Autodesk Fusion 360 part; units mm, degrees
note: some values were not read from the file. Chosen so that the rebuilt part matches the saved one: a direction. Set by a fixed rule: which sketch regions a step uses.
(part 3 of 6)
  spline S31 degree 5 poles (7.4784, -26.4341) (7.4757, -26.4291) (7.4705, -26.4191) (7.463, -26.4039) (7.4538, -26.3832) (7.4432, -26.357) (7.4334, -26.3303) (7.4239, -26.3035) (7.4148, -26.2765) (7.4058, -26.2495) (7.3969, -26.2223) (7.3883, -26.1951) (7.38, -26.1677) (7.3721, -26.1402) (7.3644, -26.1125) (7.3571, -26.0846) (7.3501, -26.0566) (7.3434, -26.0285) (7.3368, -26.0003) (7.3304, -25.9721) (7.3243, -25.9437) (7.3183, -25.9153) (7.3126, -25.8867) (7.307, -25.8581) (7.3017, -25.8294) (7.2966, -25.8006) (7.2917, -25.7717) (7.287, -25.7427) (7.2825, -25.7137) (7.2782, -25.6845) (7.2741, -25.6553) (7.2701, -25.6261) (7.2663, -25.5967) (7.2627, -25.5673) (7.2593, -25.5379) (7.256, -25.5083) (7.253, -25.4787) (7.2501, -25.4491) (7.2474, -25.4193) (7.2448, -25.3895) (7.2424, -25.3597) (7.2402, -25.3298) (7.2381, -25.2998) (7.2362, -25.2698) (7.2345, -25.2397) (7.2329, -25.2096) (7.2315, -25.1794) (7.2302, -25.1492) (7.2291, -25.1189) (7.2282, -25.0885) (7.2274, -25.0581) (7.2267, -25.0277) (7.2263, -24.9972) (7.2259, -24.9667) (7.2257, -24.9361) (7.2257, -24.9055) (7.2258, -24.8748) (7.2261, -24.8441) (7.2265, -24.8134) (7.227, -24.7826) (7.2278, -24.7517) (7.2286, -24.7208) (7.2296, -24.6899) (7.2307, -24.659) (7.232, -24.628) (7.2335, -24.5969) (7.235, -24.5659) (7.2367, -24.5348) (7.2386, -24.5036) (7.2406, -24.4724) (7.2427, -24.4412) (7.2445, -24.4162) (7.2459, -24.3975) (7.2469, -24.3849) (7.2474, -24.3787) knots 0 0 0 0 0 0 0.01428571 0.02857143 0.04285714 0.05714286 0.07142857 0.08571429 0.1 0.11428571 0.12857143 0.14285714 0.15714286 0.17142857 0.18571429 0.2 0.21428571 0.22857143 0.24285714 0.25714286 0.27142857 0.28571429 0.3 0.31428571 0.32857143 0.34285714 0.35714286 0.37142857 0.38571429 0.4 0.41428571 0.42857143 0.44285714 0.45714286 0.47142857 0.48571429 0.5 0.51428571 0.52857143 0.54285714 0.55714286 0.57142857 0.58571429 0.6 0.61428571 0.62857143 0.64285714 0.65714286 0.67142857 0.68571429 0.7 0.71428571 0.72857143 0.74285714 0.75714286 0.77142857 0.78571429 0.8 0.81428571 0.82857143 0.84285714 0.85714286 0.87142857 0.88571429 0.9 0.91428571 0.92857143 0.94285714 0.95714286 0.97142857 0.98571429 1 1 1 1 1 1
  line L31 (7.4784, -26.4341) -> (7.7091, -26.8632)
  arc A63 (7.6692, -26.9982) -> (7.7091, -26.8632) centre (7.621, -26.9106) ccw
  arc A64 (7.6692, -26.9982) -> (6.7944, -27.5287) centre (13.5, -37.5997) ccw
  arc A65 (6.6562, -27.5017) -> (6.7944, -27.5287) centre (6.7389, -27.4455) ccw
  line L32 (6.6562, -27.5017) -> (6.3823, -27.0988)
  spline S32 degree 5 poles (6.3823, -27.0988) (6.3792, -27.0941) (6.3727, -27.0848) (6.3626, -27.0712) (6.3486, -27.0534) (6.3302, -27.0319) (6.3112, -27.0109) (6.2917, -26.9901) (6.2721, -26.9695) (6.2522, -26.949) (6.2322, -26.9287) (6.2121, -26.9084) (6.1916, -26.8884) (6.1709, -26.8686) (6.1498, -26.849) (6.1285, -26.8297) (6.1069, -26.8105) (6.0851, -26.7916) (6.0632, -26.7727) (6.041, -26.754) (6.0188, -26.7354) (5.9963, -26.717) (5.9736, -26.6987) (5.9508, -26.6806) (5.9278, -26.6626) (5.9046, -26.6447) (5.8812, -26.627) (5.8577, -26.6095) (5.8341, -26.5921) (5.8102, -26.5748) (5.7863, -26.5576) (5.7621, -26.5405) (5.7379, -26.5236) (5.7135, -26.5068) (5.6889, -26.4902) (5.6642, -26.4737) (5.6394, -26.4573) (5.6144, -26.441) (5.5893, -26.4248) (5.5641, -26.4088) (5.5387, -26.3929) (5.5132, -26.3771) (5.4876, -26.3614) (5.4619, -26.3458) (5.436, -26.3304) (5.41, -26.315) (5.3839, -26.2998) (5.3577, -26.2847) (5.3313, -26.2698) (5.3048, -26.2549) (5.2783, -26.2401) (5.2516, -26.2255) (5.2248, -26.211) (5.1978, -26.1966) (5.1708, -26.1823) (5.1437, -26.1681) (5.1164, -26.154) (5.0891, -26.1401) (5.0616, -26.1262) (5.034, -26.1125) (5.0064, -26.0988) (4.9786, -26.0853) (4.9507, -26.0719) (4.9227, -26.0586) (4.8947, -26.0454) (4.8665, -26.0323) (4.8382, -26.0194) (4.8098, -26.0065) (4.7814, -25.9937) (4.7528, -25.9811) (4.7241, -25.9686) (4.7011, -25.9586) (4.6838, -25.9512) (4.6723, -25.9463) (4.6665, -25.9438) knots 0 0 0 0 0 0 0.01428571 0.02857143 0.04285714 0.05714286 0.07142857 0.08571429 0.1 0.11428571 0.12857143 0.14285714 0.15714286 0.17142857 0.18571429 0.2 0.21428571 0.22857143 0.24285714 0.25714286 0.27142857 0.28571429 0.3 0.31428571 0.32857143 0.34285714 0.35714286 0.37142857 0.38571429 0.4 0.41428571 0.42857143 0.44285714 0.45714286 0.47142857 0.48571429 0.5 0.51428571 0.52857143 0.54285714 0.55714286 0.57142857 0.58571429 0.6 0.61428571 0.62857143 0.64285714 0.65714286 0.67142857 0.68571429 0.7 0.71428571 0.72857143 0.74285714 0.75714286 0.77142857 0.78571429 0.8 0.81428571 0.82857143 0.84285714 0.85714286 0.87142857 0.88571429 0.9 0.91428571 0.92857143 0.94285714 0.95714286 0.97142857 0.98571429 1 1 1 1 1 1
  arc A66 (4.6665, -25.9438) -> (4.0386, -26.4475) centre (13.5, -37.5997) ccw
  spline S33 degree 5 poles (4.7937, -28.373) (4.7898, -28.3689) (4.7822, -28.3606) (4.771, -28.3478) (4.7568, -28.3303) (4.7398, -28.3077) (4.7233, -28.2845) (4.7073, -28.261) (4.6915, -28.2373) (4.6758, -28.2135) (4.6602, -28.1896) (4.6449, -28.1655) (4.6297, -28.1412) (4.6149, -28.1167) (4.6004, -28.0919) (4.5861, -28.0669) (4.5721, -28.0416) (4.5583, -28.0163) (4.5447, -27.9907) (4.5312, -27.9651) (4.5179, -27.9393) (4.5048, -27.9133) (4.4918, -27.8873) (4.4791, -27.8611) (4.4665, -27.8347) (4.4542, -27.8082) (4.442, -27.7815) (4.4299, -27.7548) (4.418, -27.7279) (4.4063, -27.7009) (4.3948, -27.6737) (4.3834, -27.6465) (4.3721, -27.6191) (4.361, -27.5917) (4.3501, -27.5641) (4.3393, -27.5364) (4.3287, -27.5086) (4.3182, -27.4807) (4.3079, -27.4527) (4.2977, -27.4245) (4.2877, -27.3963) (4.2778, -27.368) (4.268, -27.3396) (4.2584, -27.3111) (4.249, -27.2825) (4.2396, -27.2538) (4.2305, -27.225) (4.2214, -27.1961) (4.2125, -27.1672) (4.2037, -27.1381) (4.1951, -27.109) (4.1866, -27.0797) (4.1783, -27.0504) (4.17, -27.021) (4.1619, -26.9915) (4.154, -26.9619) (4.1462, -26.9323) (4.1385, -26.9026) (4.1309, -26.8727) (4.1235, -26.8428) (4.1162, -26.8129) (4.109, -26.7828) (4.102, -26.7527) (4.095, -26.7225) (4.0883, -26.6922) (4.0816, -26.6619) (4.0751, -26.6315) (4.0687, -26.601) (4.0624, -26.5704) (4.0563, -26.5398) (4.0502, -26.5091) (4.0455, -26.4845) (4.0421, -26.466) (4.0398, -26.4536) (4.0386, -26.4475) knots 0 0 0 0 0 0 0.01428571 0.02857143 0.04285714 0.05714286 0.07142857 0.08571429 0.1 0.11428571 0.12857143 0.14285714 0.15714286 0.17142857 0.18571429 0.2 0.21428571 0.22857143 0.24285714 0.25714286 0.27142857 0.28571429 0.3 0.31428571 0.32857143 0.34285714 0.35714286 0.37142857 0.38571429 0.4 0.41428571 0.42857143 0.44285714 0.45714286 0.47142857 0.48571429 0.5 0.51428571 0.52857143 0.54285714 0.55714286 0.57142857 0.58571429 0.6 0.61428571 0.62857143 0.64285714 0.65714286 0.67142857 0.68571429 0.7 0.71428571 0.72857143 0.74285714 0.75714286 0.77142857 0.78571429 0.8 0.81428571 0.82857143 0.84285714 0.85714286 0.87142857 0.88571429 0.9 0.91428571 0.92857143 0.94285714 0.95714286 0.97142857 0.98571429 1 1 1 1 1 1
  line L33 (4.7937, -28.373) -> (5.1276, -28.7278)
  arc A67 (5.124, -28.8685) -> (5.1276, -28.7278) centre (5.0548, -28.7964) ccw
  arc A68 (5.124, -28.8685) -> (4.4163, -29.6074) centre (13.5, -37.5997) ccw
  arc A69 (4.2759, -29.6171) -> (4.4163, -29.6074) centre (4.3412, -29.5414) ccw
  line L34 (4.2759, -29.6171) -> (3.907, -29.2988)
  spline S34 degree 5 poles (3.907, -29.2988) (3.9027, -29.2951) (3.8941, -29.2878) (3.8809, -29.2772) (3.8627, -29.2637) (3.8394, -29.2477) (3.8155, -29.2323) (3.7914, -29.2173) (3.767, -29.2025) (3.7426, -29.1878) (3.718, -29.1733) (3.6933, -29.159) (3.6683, -29.1449) (3.6432, -29.1312) (3.6178, -29.1177) (3.5922, -29.1046) (3.5664, -29.0916) (3.5404, -29.0789) (3.5143, -29.0664) (3.4881, -29.0541) (3.4618, -29.0419) (3.4353, -29.0299) (3.4087, -29.0181) (3.382, -29.0065) (3.3551, -28.9951) (3.3281, -28.9838) (3.3009, -28.9728) (3.2736, -28.9619) (3.2463, -28.9512) (3.2188, -28.9407) (3.1912, -28.9303) (3.1635, -28.9201) (3.1357, -28.91) (3.1077, -28.9001) (3.0797, -28.8904) (3.0516, -28.8808) (3.0233, -28.8714) (2.995, -28.8621) (2.9666, -28.853) (2.9381, -28.8441) (2.9094, -28.8353) (2.8807, -28.8266) (2.8519, -28.8181) (2.823, -28.8097) (2.794, -28.8015) (2.765, -28.7934) (2.7358, -28.7855) (2.7066, -28.7777) (2.6772, -28.77) (2.6478, -28.7625) (2.6183, -28.7551) (2.5888, -28.7479) (2.5591, -28.7408) (2.5294, -28.7339) (2.4996, -28.7271) (2.4697, -28.7204) (2.4397, -28.7138) (2.4097, -28.7074) (2.3796, -28.7012) (2.3494, -28.695) (2.3191, -28.689) (2.2888, -28.6832) (2.2584, -28.6774) (2.2279, -28.6718) (2.1974, -28.6663) (2.1668, -28.661) (2.1361, -28.6558) (2.1054, -28.6507) (2.0746, -28.6458) (2.0437, -28.6409) (2.0128, -28.6362) (1.988, -28.6326) (1.9694, -28.6299) (1.9569, -28.6282) (1.9507, -28.6273) knots 0 0 0 0 0 0 0.01428571 0.02857143 0.04285714 0.05714286 0.07142857 0.08571429 0.1 0.11428571 0.12857143 0.14285714 0.15714286 0.17142857 0.18571429 0.2 0.21428571 0.22857143 0.24285714 0.25714286 0.27142857 0.28571429 0.3 0.31428571 0.32857143 0.34285714 0.35714286 0.37142857 0.38571429 0.4 0.41428571 0.42857143 0.44285714 0.45714286 0.47142857 0.48571429 0.5 0.51428571 0.52857143 0.54285714 0.55714286 0.57142857 0.58571429 0.6 0.61428571 0.62857143 0.64285714 0.65714286 0.67142857 0.68571429 0.7 0.71428571 0.72857143 0.74285714 0.75714286 0.77142857 0.78571429 0.8 0.81428571 0.82857143 0.84285714 0.85714286 0.87142857 0.88571429 0.9 0.91428571 0.92857143 0.94285714 0.95714286 0.97142857 0.98571429 1 1 1 1 1 1
  arc A70 (1.9507, -28.6273) -> (1.4746, -29.2762) centre (13.5, -37.5997) ccw
  spline S35 degree 5 poles (2.7023, -30.9408) (2.6975, -30.9378) (2.688, -30.9317) (2.6739, -30.9223) (2.6556, -30.9091) (2.6333, -30.8916) (2.6114, -30.8735) (2.5899, -30.8549) (2.5685, -30.8362) (2.5471, -30.8172) (2.5259, -30.7982) (2.5048, -30.7789) (2.4839, -30.7593) (2.4633, -30.7394) (2.4428, -30.7192) (2.4226, -30.6988) (2.4025, -30.678) (2.3826, -30.6571) (2.3628, -30.636) (2.3432, -30.6147) (2.3237, -30.5932) (2.3043, -30.5715) (2.285, -30.5497) (2.2659, -30.5277) (2.247, -30.5054) (2.2281, -30.483) (2.2095, -30.4605) (2.1909, -30.4377) (2.1725, -30.4148) (2.1542, -30.3918) (2.136, -30.3686) (2.1179, -30.3452) (2.1, -30.3217) (2.0822, -30.298) (2.0645, -30.2742) (2.0469, -30.2502) (2.0294, -30.2261) (2.0121, -30.2019) (1.9949, -30.1775) (1.9777, -30.153) (1.9607, -30.1283) (1.9439, -30.1035) (1.9271, -30.0786) (1.9104, -30.0536) (1.8939, -30.0284) (1.8775, -30.0031) (1.8611, -29.9777) (1.8449, -29.9521) (1.8288, -29.9264) (1.8128, -29.9006) (1.797, -29.8747) (1.7812, -29.8487) (1.7655, -29.8225) (1.75, -29.7962) (1.7345, -29.7698) (1.7192, -29.7433) (1.7039, -29.7167) (1.6888, -29.69) (1.6738, -29.6632) (1.6589, -29.6362) (1.6441, -29.6091) (1.6294, -29.582) (1.6148, -29.5547) (1.6003, -29.5273) (1.5859, -29.4998) (1.5716, -29.4722) (1.5574, -29.4446) (1.5434, -29.4168) (1.5294, -29.3889) (1.5155, -29.3609) (1.5018, -29.3328) (1.4908, -29.3102) (1.4827, -29.2932) (1.4773, -29.2819) (1.4746, -29.2762) knots 0 0 0 0 0 0 0.01428571 0.02857143 0.04285714 0.05714286 0.07142857 0.08571429 0.1 0.11428571 0.12857143 0.14285714 0.15714286 0.17142857 0.18571429 0.2 0.21428571 0.22857143 0.24285714 0.25714286 0.27142857 0.28571429 0.3 0.31428571 0.32857143 0.34285714 0.35714286 0.37142857 0.38571429 0.4 0.41428571 0.42857143 0.44285714 0.45714286 0.47142857 0.48571429 0.5 0.51428571 0.52857143 0.54285714 0.55714286 0.57142857 0.58571429 0.6 0.61428571 0.62857143 0.64285714 0.65714286 0.67142857 0.68571429 0.7 0.71428571 0.72857143 0.74285714 0.75714286 0.77142857 0.78571429 0.8 0.81428571 0.82857143 0.84285714 0.85714286 0.87142857 0.88571429 0.9 0.91428571 0.92857143 0.94285714 0.95714286 0.97142857 0.98571429 1 1 1 1 1 1
  line L35 (2.7023, -30.9408) -> (3.1167, -31.1971)
  arc A71 (3.1496, -31.3339) -> (3.1167, -31.1971) centre (3.0641, -31.2821) ccw
  arc A72 (3.1496, -31.3339) -> (2.6572, -32.2308) centre (13.5, -37.5997) ccw
  arc A73 (2.5241, -32.2765) -> (2.6572, -32.2308) centre (2.5676, -32.1864) ccw
  line L36 (2.5241, -32.2765) -> (2.0855, -32.0645)
  spline S36 degree 5 poles (2.0855, -32.0645) (2.0804, -32.062) (2.0701, -32.0572) (2.0546, -32.0504) (2.0336, -32.042) (2.0069, -32.0326) (1.9799, -32.0239) (1.9527, -32.0157) (1.9253, -32.0077) (1.8979, -31.9998) (1.8704, -31.9922) (1.8428, -31.9848) (1.8151, -31.9776) (1.7872, -31.9709) (1.7592, -31.9644) (1.7311, -31.9584) (1.7028, -31.9526) (1.6745, -31.947) (1.646, -31.9417) (1.6175, -31.9365) (1.5889, -31.9316) (1.5602, -31.9268) (1.5315, -31.9223) (1.5026, -31.918) (1.4737, -31.914) (1.4447, -31.9101) (1.4156, -31.9065) (1.3865, -31.903) (1.3573, -31.8998) (1.328, -31.8967) (1.2986, -31.8938) (1.2692, -31.8911) (1.2398, -31.8886) (1.2102, -31.8863) (1.1806, -31.8841) (1.151, -31.8822) (1.1213, -31.8804) (1.0915, -31.8788) (1.0617, -31.8773) (1.0318, -31.876) (1.0019, -31.8749) (0.9719, -31.874) (0.9419, -31.8732) (0.9118, -31.8726) (0.8817, -31.8722) (0.8515, -31.8719) (0.8213, -31.8718) (0.791, -31.8718) (0.7607, -31.872) (0.7304, -31.8724) (0.7, -31.8729) (0.6695, -31.8736) (0.6391, -31.8744) (0.6085, -31.8754) (0.578, -31.8765) (0.5474, -31.8778) (0.5168, -31.8792) (0.4861, -31.8808) (0.4554, -31.8826) (0.4246, -31.8844) (0.3939, -31.8865) (0.363, -31.8887) (0.3322, -31.891) (0.3013, -31.8934) (0.2704, -31.8961) (0.2395, -31.8988) (0.2085, -31.9017) (0.1775, -31.9048) (0.1464, -31.908) (0.1154, -31.9113) (0.0843, -31.9148) (0.0594, -31.9177) (0.0407, -31.9199) (0.0282, -31.9214) (0.022, -31.9222) knots 0 0 0 0 0 0 0.01428571 0.02857143 0.04285714 0.05714286 0.07142857 0.08571429 0.1 0.11428571 0.12857143 0.14285714 0.15714286 0.17142857 0.18571429 0.2 0.21428571 0.22857143 0.24285714 0.25714286 0.27142857 0.28571429 0.3 0.31428571 0.32857143 0.34285714 0.35714286 0.37142857 0.38571429 0.4 0.41428571 0.42857143 0.44285714 0.45714286 0.47142857 0.48571429 0.5 0.51428571 0.52857143 0.54285714 0.55714286 0.57142857 0.58571429 0.6 0.61428571 0.62857143 0.64285714 0.65714286 0.67142857 0.68571429 0.7 0.71428571 0.72857143 0.74285714 0.75714286 0.77142857 0.78571429 0.8 0.81428571 0.82857143 0.84285714 0.85714286 0.87142857 0.88571429 0.9 0.91428571 0.92857143 0.94285714 0.95714286 0.97142857 0.98571429 1 1 1 1 1 1
  arc A74 (0.022, -31.9222) -> (-0.2699, -32.6723) centre (13.5, -37.5997) ccw
  spline S37 degree 5 poles (1.3468, -33.9623) (1.3414, -33.9607) (1.3306, -33.9573) (1.3146, -33.9518) (1.2934, -33.9438) (1.2674, -33.9327) (1.2416, -33.9208) (1.216, -33.9085) (1.1904, -33.8959) (1.1649, -33.8832) (1.1395, -33.8702) (1.1141, -33.857) (1.0889, -33.8435) (1.0638, -33.8297) (1.0388, -33.8155) (1.0139, -33.8009) (0.9892, -33.7861) (0.9645, -33.771) (0.94, -33.7557) (0.9155, -33.7403) (0.8911, -33.7246) (0.8667, -33.7087) (0.8425, -33.6926) (0.8183, -33.6762) (0.7943, -33.6597) (0.7703, -33.6429) (0.7464, -33.6259) (0.7226, -33.6088) (0.6989, -33.5914) (0.6752, -33.5739) (0.6516, -33.5562) (0.6281, -33.5383) (0.6047, -33.5202) (0.5814, -33.502) (0.5581, -33.4835) (0.535, -33.465) (0.5119, -33.4462) (0.4888, -33.4273) (0.4659, -33.4082) (0.443, -33.3889) (0.4202, -33.3695) (0.3975, -33.3499) (0.3748, -33.3302) (0.3523, -33.3103) (0.3298, -33.2903) (0.3073, -33.2701) (0.285, -33.2497) (0.2627, -33.2292) (0.2405, -33.2086) (0.2184, -33.1878) (0.1964, -33.1669) (0.1744, -33.1458) (0.1525, -33.1246) (0.1307, -33.1033) (0.1089, -33.0818) (0.0872, -33.0601) (0.0656, -33.0384) (0.0441, -33.0165) (0.0226, -32.9944) (0.0013, -32.9723) (-0.0201, -32.95) (-0.0413, -32.9275) (-0.0624, -32.905) (-0.0835, -32.8823) (-0.1045, -32.8594) (-0.1255, -32.8365) (-0.1463, -32.8134) (-0.1671, -32.7902) (-0.1878, -32.7669) (-0.2085, -32.7434) (-0.229, -32.7198) (-0.2454, -32.7009) (-0.2577, -32.6866) (-0.2659, -32.677) (-0.2699, -32.6723) knots 0 0 0 0 0 0 0.01428571 0.02857143 0.04285714 0.05714286 0.07142857 0.08571429 0.1 0.11428571 0.12857143 0.14285714 0.15714286 0.17142857 0.18571429 0.2 0.21428571 0.22857143 0.24285714 0.25714286 0.27142857 0.28571429 0.3 0.31428571 0.32857143 0.34285714 0.35714286 0.37142857 0.38571429 0.4 0.41428571 0.42857143 0.44285714 0.45714286 0.47142857 0.48571429 0.5 0.51428571 0.52857143 0.54285714 0.55714286 0.57142857 0.58571429 0.6 0.61428571 0.62857143 0.64285714 0.65714286 0.67142857 0.68571429 0.7 0.71428571 0.72857143 0.74285714 0.75714286 0.77142857 0.78571429 0.8 0.81428571 0.82857143 0.84285714 0.85714286 0.87142857 0.88571429 0.9 0.91428571 0.92857143 0.94285714 0.95714286 0.97142857 0.98571429 1 1 1 1 1 1
  line L37 (1.3468, -33.9623) -> (1.8134, -34.1026)
  arc A75 (1.8806, -34.2263) -> (1.8134, -34.1026) centre (1.7846, -34.1984) ccw
  arc A76 (1.8806, -34.2263) -> (1.6371, -35.2201) centre (13.5, -37.5997) ccw
  arc A77 (1.5204, -35.2986) -> (1.6371, -35.2201) centre (1.5391, -35.2004) ccw
  line L38 (1.5204, -35.2986) -> (1.0418, -35.2074)
  spline S38 degree 5 poles (1.0418, -35.2074) (1.0362, -35.2063) (1.0251, -35.2043) (1.0083, -35.2018) (0.9859, -35.1992) (0.9576, -35.1969) (0.9293, -35.1955) (0.9009, -35.1946) (0.8724, -35.194) (0.8439, -35.1935) (0.8153, -35.1932) (0.7868, -35.1932) (0.7581, -35.1935) (0.7295, -35.1941) (0.7008, -35.1952) (0.672, -35.1966) (0.6432, -35.1983) (0.6144, -35.2003) (0.5855, -35.2025) (0.5566, -35.2049) (0.5277, -35.2075) (0.4988, -35.2104) (0.4699, -35.2135) (0.4409, -35.2168) (0.4119, -35.2203) (0.3829, -35.2241) (0.3539, -35.2281) (0.3248, -35.2324) (0.2958, -35.2368) (0.2667, -35.2414) (0.2376, -35.2462) (0.2085, -35.2512) (0.1794, -35.2564) (0.1502, -35.2618) (0.1211, -35.2674) (0.092, -35.2731) (0.0628, -35.2791) (0.0336, -35.2852) (0.0044, -35.2916) (-0.0247, -35.2981) (-0.0539, -35.3048) (-0.0831, -35.3116) (-0.1123, -35.3186) (-0.1415, -35.3258) (-0.1708, -35.3332) (-0.2, -35.3407) (-0.2292, -35.3484) (-0.2584, -35.3563) (-0.2876, -35.3644) (-0.3169, -35.3726) (-0.3461, -35.3809) (-0.3753, -35.3895) (-0.4045, -35.3981) (-0.4338, -35.407) (-0.463, -35.416) (-0.4922, -35.4251) (-0.5214, -35.4345) (-0.5506, -35.4439) (-0.5798, -35.4536) (-0.6091, -35.4633) (-0.6383, -35.4733) (-0.6675, -35.4833) (-0.6967, -35.4936) (-0.7258, -35.504) (-0.755, -35.5145) (-0.7842, -35.5252) (-0.8134, -35.536) (-0.8425, -35.547) (-0.8717, -35.5581) (-0.9008, -35.5693) (-0.93, -35.5807) (-0.9533, -35.59) (-0.9707, -35.597) (-0.9824, -35.6016) (-0.9882, -35.604) knots 0 0 0 0 0 0 0.01428571 0.02857143 0.04285714 0.05714286 0.07142857 0.08571429 0.1 0.11428571 0.12857143 0.14285714 0.15714286 0.17142857 0.18571429 0.2 0.21428571 0.22857143 0.24285714 0.25714286 0.27142857 0.28571429 0.3 0.31428571 0.32857143 0.34285714 0.35714286 0.37142857 0.38571429 0.4 0.41428571 0.42857143 0.44285714 0.45714286 0.47142857 0.48571429 0.5 0.51428571 0.52857143 0.54285714 0.55714286 0.57142857 0.58571429 0.6 0.61428571 0.62857143 0.64285714 0.65714286 0.67142857 0.68571429 0.7 0.71428571 0.72857143 0.74285714 0.75714286 0.77142857 0.78571429 0.8 0.81428571 0.82857143 0.84285714 0.85714286 0.87142857 0.88571429 0.9 0.91428571 0.92857143 0.94285714 0.95714286 0.97142857 0.98571429 1 1 1 1 1 1
  arc A78 (-0.9882, -35.604) -> (-1.076, -36.4041) centre (13.5, -37.5997) ccw
  spline S39 degree 5 poles (0.8195, -37.2317) (0.8138, -37.2316) (0.8025, -37.2311) (0.7856, -37.2299) (0.7631, -37.2276) (0.7351, -37.2237) (0.7071, -37.2189) (0.6792, -37.2136) (0.6512, -37.2081) (0.6233, -37.2024) (0.5954, -37.1964) (0.5675, -37.1903) (0.5396, -37.1838) (0.5118, -37.1769) (0.484, -37.1696) (0.4562, -37.162) (0.4284, -37.1541) (0.4007, -37.1459) (0.373, -37.1375) (0.3454, -37.1289) (0.3177, -37.12) (0.2901, -37.111) (0.2625, -37.1017) (0.235, -37.0922) (0.2075, -37.0824) (0.18, -37.0724) (0.1525, -37.0622) (0.125, -37.0518) (0.0976, -37.0412) (0.0703, -37.0304) (0.0429, -37.0194) (0.0156, -37.0082) (-0.0117, -36.9968) (-0.039, -36.9852) (-0.0662, -36.9734) (-0.0934, -36.9614) (-0.1206, -36.9493) (-0.1477, -36.937) (-0.1749, -36.9245) (-0.2019, -36.9118) (-0.229, -36.8989) (-0.256, -36.8859) (-0.283, -36.8727) (-0.3099, -36.8593) (-0.3368, -36.8458) (-0.3637, -36.8321) (-0.3906, -36.8182) (-0.4174, -36.8042) (-0.4442, -36.79) (-0.4709, -36.7757) (-0.4976, -36.7612) (-0.5243, -36.7465) (-0.551, -36.7317) (-0.5776, -36.7167) (-0.6041, -36.7016) (-0.6307, -36.6863) (-0.6572, -36.6709) (-0.6836, -36.6553) (-0.7101, -36.6396) (-0.7365, -36.6237) (-0.7628, -36.6076) (-0.7891, -36.5915) (-0.8154, -36.5751) (-0.8417, -36.5587) (-0.8679, -36.5421) (-0.894, -36.5253) (-0.9201, -36.5084) (-0.9462, -36.4914) (-0.9723, -36.4742) (-0.9983, -36.4569) (-1.0242, -36.4394) (-1.045, -36.4254) (-1.0605, -36.4148) (-1.0709, -36.4076) (-1.076, -36.4041) knots 0 0 0 0 0 0 0.01428571 0.02857143 0.04285714 0.05714286 0.07142857 0.08571429 0.1 0.11428571 0.12857143 0.14285714 0.15714286 0.17142857 0.18571429 0.2 0.21428571 0.22857143 0.24285714 0.25714286 0.27142857 0.28571429 0.3 0.31428571 0.32857143 0.34285714 0.35714286 0.37142857 0.38571429 0.4 0.41428571 0.42857143 0.44285714 0.45714286 0.47142857 0.48571429 0.5 0.51428571 0.52857143 0.54285714 0.55714286 0.57142857 0.58571429 0.6 0.61428571 0.62857143 0.64285714 0.65714286 0.67142857 0.68571429 0.7 0.71428571 0.72857143 0.74285714 0.75714286 0.77142857 0.78571429 0.8 0.81428571 0.82857143 0.84285714 0.85714286 0.87142857 0.88571429 0.9 0.91428571 0.92857143 0.94285714 0.95714286 0.97142857 0.98571429 1 1 1 1 1 1
  line L39 (0.8195, -37.2317) -> (1.3065, -37.2465)
  arc A79 (1.4034, -37.3486) -> (1.3065, -37.2465) centre (1.3034, -37.3465) ccw
  arc A80 (1.4034, -37.3486) -> (1.4254, -38.3715) centre (13.5, -37.5997) ccw
  arc A81 (1.333, -38.4776) -> (1.4254, -38.3715) centre (1.3256, -38.3779) ccw
  line L40 (1.333, -38.4776) -> (0.8471, -38.5133)
  spline S40 degree 5 poles (0.8471, -38.5133) (0.8414, -38.5137) (0.8302, -38.5147) (0.8133, -38.5166) (0.791, -38.5198) (0.7631, -38.525) (0.7354, -38.531) (0.7077, -38.5375) (0.68, -38.5442) (0.6524, -38.5511) (0.6247, -38.5582) (0.5971, -38.5656) (0.5695, -38.5733) (0.542, -38.5814) (0.5145, -38.5898) (0.4871, -38.5986) (0.4598, -38.6077) (0.4324, -38.6171) (0.4051, -38.6267) (0.3779, -38.6365) (0.3506, -38.6465) (0.3234, -38.6568) (0.2963, -38.6672) (0.2691, -38.6779) (0.2421, -38.6889) (0.215, -38.7) (0.188, -38.7114) (0.161, -38.723) (0.1341, -38.7348) (0.1072, -38.7468) (0.0804, -38.7589) (0.0535, -38.7713) (0.0268, -38.7839) (0, -38.7966) (-0.0267, -38.8096) (-0.0533, -38.8227) (-0.08, -38.836) (-0.1066, -38.8495) (-0.1331, -38.8631) (-0.1596, -38.877) (-0.1861, -38.891) (-0.2125, -38.9051) (-0.2389, -38.9195) (-0.2652, -38.934) (-0.2916, -38.9487) (-0.3178, -38.9635) (-0.344, -38.9785) (-0.3702, -38.9937) (-0.3964, -39.009) (-0.4225, -39.0245) (-0.4486, -39.0402) (-0.4746, -39.056) (-0.5006, -39.0719) (-0.5265, -39.088) (-0.5524, -39.1043) (-0.5782, -39.1207) (-0.6041, -39.1373) (-0.6298, -39.154) (-0.6556, -39.1708) (-0.6812, -39.1878) (-0.7069, -39.205) (-0.7325, -39.2223) (-0.758, -39.2397) (-0.7835, -39.2573) (-0.809, -39.275) (-0.8344, -39.2929) (-0.8598, -39.3109) (-0.8851, -39.329) (-0.9104, -39.3473) (-0.9356, -39.3657) (-0.9608, -39.3843) (-0.9809, -39.3992) (-0.996, -39.4105) (-1.006, -39.418) (-1.011, -39.4218) knots 0 0 0 0 0 0 0.01428571 0.02857143 0.04285714 0.05714286 0.07142857 0.08571429 0.1 0.11428571 0.12857143 0.14285714 0.15714286 0.17142857 0.18571429 0.2 0.21428571 0.22857143 0.24285714 0.25714286 0.27142857 0.28571429 0.3 0.31428571 0.32857143 0.34285714 0.35714286 0.37142857 0.38571429 0.4 0.41428571 0.42857143 0.44285714 0.45714286 0.47142857 0.48571429 0.5 0.51428571 0.52857143 0.54285714 0.55714286 0.57142857 0.58571429 0.6 0.61428571 0.62857143 0.64285714 0.65714286 0.67142857 0.68571429 0.7 0.71428571 0.72857143 0.74285714 0.75714286 0.77142857 0.78571429 0.8 0.81428571 0.82857143 0.84285714 0.85714286 0.87142857 0.88571429 0.9 0.91428571 0.92857143 0.94285714 0.95714286 0.97142857 0.98571429 1 1 1 1 1 1
  arc A82 (-1.011, -39.4218) -> (-0.8888, -40.2174) centre (13.5, -37.5997) ccw
  spline S41 degree 5 poles (1.1563, -40.5262) (1.1508, -40.5275) (1.1398, -40.53) (1.1231, -40.5333) (1.1008, -40.5369) (1.0727, -40.5403) (1.0445, -40.5429) (1.0161, -40.5451) (0.9877, -40.5469) (0.9592, -40.5486) (0.9307, -40.5501) (0.9022, -40.5514) (0.8736, -40.5523) (0.8449, -40.5529) (0.8162, -40.5531) (0.7874, -40.5529) (0.7585, -40.5525) (0.7296, -40.5517) (0.7007, -40.5508) (0.6718, -40.5496) (0.6428, -40.5482) (0.6138, -40.5466) (0.5847, -40.5448) (0.5556, -40.5427) (0.5265, -40.5404) (0.4974, -40.5379) (0.4682, -40.5351) (0.439, -40.5322) (0.4097, -40.529) (0.3805, -40.5256) (0.3512, -40.5221) (0.3219, -40.5183) (0.2926, -40.5144) (0.2633, -40.5103) (0.2339, -40.5059) (0.2046, -40.5014) (0.1752, -40.4967) (0.1458, -40.4918) (0.1163, -40.4868) (0.0869, -40.4815) (0.0574, -40.4761) (0.028, -40.4705) (-0.0015, -40.4648) (-0.031, -40.4588) (-0.0605, -40.4527) (-0.09, -40.4465) (-0.1195, -40.44) (-0.1491, -40.4334) (-0.1786, -40.4266) (-0.2082, -40.4197) (-0.2377, -40.4126) (-0.2673, -40.4053) (-0.2968, -40.3979) (-0.3264, -40.3903) (-0.356, -40.3826) (-0.3856, -40.3747) (-0.4152, -40.3667) (-0.4448, -40.3585) (-0.4744, -40.3501) (-0.504, -40.3416) (-0.5336, -40.3329) (-0.5632, -40.3241) (-0.5928, -40.3152) (-0.6224, -40.306) (-0.652, -40.2968) (-0.6816, -40.2874) (-0.7112, -40.2778) (-0.7408, -40.2681) (-0.7704, -40.2583) (-0.8, -40.2483) (-0.8296, -40.2381) (-0.8533, -40.2299) (-0.8711, -40.2237) (-0.8829, -40.2195) (-0.8888, -40.2174) knots 0 0 0 0 0 0 0.01428571 0.02857143 0.04285714 0.05714286 0.07142857 0.08571429 0.1 0.11428571 0.12857143 0.14285714 0.15714286 0.17142857 0.18571429 0.2 0.21428571 0.22857143 0.24285714 0.25714286 0.27142857 0.28571429 0.3 0.31428571 0.32857143 0.34285714 0.35714286 0.37142857 0.38571429 0.4 0.41428571 0.42857143 0.44285714 0.45714286 0.47142857 0.48571429 0.5 0.51428571 0.52857143 0.54285714 0.55714286 0.57142857 0.58571429 0.6 0.61428571 0.62857143 0.64285714 0.65714286 0.67142857 0.68571429 0.7 0.71428571 0.72857143 0.74285714 0.75714286 0.77142857 0.78571429 0.8 0.81428571 0.82857143 0.84285714 0.85714286 0.87142857 0.88571429 0.9 0.91428571 0.92857143 0.94285714 0.95714286 0.97142857 0.98571429 1 1 1 1 1 1
  line L41 (1.1563, -40.5262) -> (1.6305, -40.4145)
  arc A83 (1.7506, -40.4879) -> (1.6305, -40.4145) centre (1.6535, -40.5118) ccw
  arc A84 (1.7506, -40.4879) -> (2.0366, -41.4703) centre (13.5, -37.5997) ccw
  arc A85 (1.9748, -41.5967) -> (2.0366, -41.4703) centre (1.9419, -41.5023) ccw
  line L42 (1.9748, -41.5967) -> (1.5147, -41.757)
  spline S42 degree 5 poles (1.5147, -41.757) (1.5093, -41.7589) (1.4987, -41.7627) (1.4829, -41.7689) (1.4622, -41.7778) (1.4366, -41.79) (1.4113, -41.803) (1.3863, -41.8164) (1.3613, -41.8301) (1.3364, -41.8439) (1.3115, -41.858) (1.2867, -41.8722) (1.2621, -41.8868) (1.2376, -41.9017) (1.2133, -41.917) (1.1891, -41.9326) (1.165, -41.9484) (1.141, -41.9646) (1.1171, -41.9809) (1.0933, -41.9974) (1.0696, -42.0142) (1.046, -42.0311) (1.0225, -42.0482) (0.999, -42.0656) (0.9757, -42.0832) (0.9525, -42.1009) (0.9293, -42.1189) (0.9063, -42.1371) (0.8833, -42.1555) (0.8604, -42.174) (0.8377, -42.1927) (0.815, -42.2116) (0.7923, -42.2307) (0.7698, -42.2499) (0.7474, -42.2693) (0.725, -42.2889) (0.7027, -42.3086) (0.6805, -42.3285) (0.6584, -42.3486) (0.6364, -42.3688) (0.6145, -42.3892) (0.5926, -42.4097) (0.5708, -42.4304) (0.5491, -42.4512) (0.5275, -42.4722) (0.506, -42.4934) (0.4845, -42.5147) (0.4632, -42.5361) (0.4419, -42.5577) (0.4207, -42.5794) (0.3995, -42.6012) (0.3785, -42.6232) (0.3575, -42.6454) (0.3366, -42.6676) (0.3158, -42.69) (0.2951, -42.7126) (0.2745, -42.7353) (0.2539, -42.7581) (0.2334, -42.781) (0.213, -42.8041) (0.1927, -42.8273) (0.1724, -42.8506) (0.1523, -42.8741) (0.1322, -42.8977) (0.1122, -42.9214) (0.0922, -42.9452) (0.0724, -42.9692) (0.0526, -42.9932) (0.0329, -43.0174) (0.0133, -43.0418) (-0.0062, -43.0662) (-0.0218, -43.0858) (-0.0334, -43.1006) (-0.0411, -43.1105) (-0.045, -43.1155) knots 0 0 0 0 0 0 0.01428571 0.02857143 0.04285714 0.05714286 0.07142857 0.08571429 0.1 0.11428571 0.12857143 0.14285714 0.15714286 0.17142857 0.18571429 0.2 0.21428571 0.22857143 0.24285714 0.25714286 0.27142857 0.28571429 0.3 0.31428571 0.32857143 0.34285714 0.35714286 0.37142857 0.38571429 0.4 0.41428571 0.42857143 0.44285714 0.45714286 0.47142857 0.48571429 0.5 0.51428571 0.52857143 0.54285714 0.55714286 0.57142857 0.58571429 0.6 0.61428571 0.62857143 0.64285714 0.65714286 0.67142857 0.68571429 0.7 0.71428571 0.72857143 0.74285714 0.75714286 0.77142857 0.78571429 0.8 0.81428571 0.82857143 0.84285714 0.85714286 0.87142857 0.88571429 0.9 0.91428571 0.92857143 0.94285714 0.95714286 0.97142857 0.98571429 1 1 1 1 1 1
  arc A86 (-0.045, -43.1155) -> (0.279, -43.8523) centre (13.5, -37.5997) ccw
  spline S43 degree 5 poles (2.3344, -43.6213) (2.3294, -43.624) (2.3194, -43.6292) (2.3041, -43.6367) (2.2835, -43.6459) (2.2572, -43.6565) (2.2306, -43.6664) (2.2038, -43.6758) (2.1768, -43.6849) (2.1498, -43.6939) (2.1226, -43.7028) (2.0954, -43.7114) (2.068, -43.7197) (2.0404, -43.7277) (2.0127, -43.7353) (1.9849, -43.7426) (1.9569, -43.7496) (1.9288, -43.7563) (1.9006, -43.7629) (1.8723, -43.7693) (1.844, -43.7754) (1.8156, -43.7814) (1.787, -43.7872) (1.7584, -43.7927) (1.7297, -43.798) (1.7009, -43.8031) (1.672, -43.808) (1.643, -43.8127) (1.6139, -43.8172) (1.5848, -43.8215) (1.5556, -43.8257) (1.5264, -43.8296) (1.497, -43.8334) (1.4676, -43.837) (1.4381, -43.8404) (1.4086, -43.8437) (1.379, -43.8467) (1.3493, -43.8496) (1.3196, -43.8524) (1.2898, -43.8549) (1.26, -43.8573) (1.2301, -43.8595) (1.2001, -43.8616) (1.1701, -43.8635) (1.14, -43.8652) (1.1099, -43.8668) (1.0797, -43.8682) (1.0494, -43.8695) (1.0191, -43.8706) (0.9888, -43.8715) (0.9584, -43.8723) (0.928, -43.873) (0.8975, -43.8735) (0.867, -43.8738) (0.8364, -43.874) (0.8058, -43.874) (0.7751, -43.8739) (0.7444, -43.8736) (0.7136, -43.8732) (0.6828, -43.8727) (0.652, -43.872) (0.6211, -43.8711) (0.5902, -43.8701) (0.5592, -43.869) (0.5283, -43.8677) (0.4972, -43.8663) (0.4661, -43.8647) (0.435, -43.863) (0.4039, -43.8611) (0.3727, -43.8591) (0.3415, -43.857) (0.3165, -43.8552) (0.2977, -43.8538) (0.2852, -43.8528) (0.279, -43.8523) knots 0 0 0 0 0 0 0.01428571 0.02857143 0.04285714 0.05714286 0.07142857 0.08571429 0.1 0.11428571 0.12857143 0.14285714 0.15714286 0.17142857 0.18571429 0.2 0.21428571 0.22857143 0.24285714 0.25714286 0.27142857 0.28571429 0.3 0.31428571 0.32857143 0.34285714 0.35714286 0.37142857 0.38571429 0.4 0.41428571 0.42857143 0.44285714 0.45714286 0.47142857 0.48571429 0.5 0.51428571 0.52857143 0.54285714 0.55714286 0.57142857 0.58571429 0.6 0.61428571 0.62857143 0.64285714 0.65714286 0.67142857 0.68571429 0.7 0.71428571 0.72857143 0.74285714 0.75714286 0.77142857 0.78571429 0.8 0.81428571 0.82857143 0.84285714 0.85714286 0.87142857 0.88571429 0.9 0.91428571 0.92857143 0.94285714 0.95714286 0.97142857 0.98571429 1 1 1 1 1 1
  line L43 (2.3344, -43.6213) -> (2.7635, -43.3906)
  arc A87 (2.8985, -43.4305) -> (2.7635, -43.3906) centre (2.8108, -43.4787) ccw
  arc A88 (2.8985, -43.4305) -> (3.429, -44.3054) centre (13.5, -37.5997) ccw
  arc A89 (3.402, -44.4435) -> (3.429, -44.3054) centre (3.3458, -44.3608) ccw
  line L44 (3.402, -44.4435) -> (2.9991, -44.7174)
  spline S44 degree 5 poles (2.9991, -44.7174) (2.9944, -44.7206) (2.9851, -44.727) (2.9714, -44.7371) (2.9537, -44.7511) (2.9322, -44.7695) (2.9111, -44.7885) (2.8904, -44.808) (2.8698, -44.8277) (2.8493, -44.8475) (2.8289, -44.8675) (2.8087, -44.8877) (2.7887, -44.9081) (2.7689, -44.9288) (2.7493, -44.9499) (2.73, -44.9712) (2.7108, -44.9928) (2.6918, -45.0146) (2.673, -45.0365) (2.6543, -45.0587) (2.6357, -45.081) (2.6173, -45.1034) (2.599, -45.1261) (2.5808, -45.1489) (2.5629, -45.1719) (2.545, -45.1951) (2.5273, -45.2185) (2.5098, -45.242) (2.4923, -45.2657) (2.475, -45.2895) (2.4579, -45.3135) (2.4408, -45.3376) (2.4239, -45.3618) (2.4071, -45.3863) (2.3905, -45.4108) (2.3739, -45.4355) (2.3575, -45.4603) (2.3413, -45.4853) (2.3251, -45.5104) (2.3091, -45.5356) (2.2931, -45.561) (2.2773, -45.5865) (2.2617, -45.6121) (2.2461, -45.6379) (2.2306, -45.6637) (2.2153, -45.6897) (2.2001, -45.7158) (2.185, -45.7421) (2.17, -45.7684) (2.1552, -45.7949) (2.1404, -45.8215) (2.1258, -45.8481) (2.1113, -45.875) (2.0969, -45.9019) (2.0826, -45.9289) (2.0684, -45.956) (2.0543, -45.9833) (2.0403, -46.0106) (2.0265, -46.0381) (2.0127, -46.0657) (1.9991, -46.0933) (1.9856, -46.1211) (1.9722, -46.149) (1.9589, -46.177) (1.9457, -46.2051) (1.9326, -46.2332) (1.9196, -46.2615) (1.9068, -46.2899) (1.894, -46.3184) (1.8814, -46.3469) (1.8688, -46.3756) (1.8589, -46.3986) (1.8515, -46.4159) (1.8466, -46.4275) (1.8441, -46.4332) knots 0 0 0 0 0 0 0.01428571 0.02857143 0.04285714 0.05714286 0.07142857 0.08571429 0.1 0.11428571 0.12857143 0.14285714 0.15714286 0.17142857 0.18571429 0.2 0.21428571 0.22857143 0.24285714 0.25714286 0.27142857 0.28571429 0.3 0.31428571 0.32857143 0.34285714 0.35714286 0.37142857 0.38571429 0.4 0.41428571 0.42857143 0.44285714 0.45714286 0.47142857 0.48571429 0.5 0.51428571 0.52857143 0.54285714 0.55714286 0.57142857 0.58571429 0.6 0.61428571 0.62857143 0.64285714 0.65714286 0.67142857 0.68571429 0.7 0.71428571 0.72857143 0.74285714 0.75714286 0.77142857 0.78571429 0.8 0.81428571 0.82857143 0.84285714 0.85714286 0.87142857 0.88571429 0.9 0.91428571 0.92857143 0.94285714 0.95714286 0.97142857 0.98571429 1 1 1 1 1 1
  arc A90 (1.8441, -46.4332) -> (2.3477, -47.0611) centre (13.5, -37.5997) ccw
  spline S45 degree 5 poles (4.2733, -46.306) (4.2692, -46.3099) (4.2609, -46.3175) (4.2481, -46.3287) (4.2306, -46.343) (4.2079, -46.36) (4.1848, -46.3764) (4.1613, -46.3924) (4.1376, -46.4082) (4.1138, -46.4239) (4.0899, -46.4395) (4.0658, -46.4549) (4.0415, -46.47) (4.0169, -46.4848) (3.9922, -46.4993) (3.9671, -46.5136) (3.9419, -46.5276) (3.9165, -46.5414) (3.891, -46.555) (3.8653, -46.5685) (3.8396, -46.5818) (3.8136, -46.5949) (3.7876, -46.6079) (3.7613, -46.6206) (3.735, -46.6332) (3.7085, -46.6456) (3.6818, -46.6578) (3.655, -46.6698) (3.6281, -46.6817) (3.6011, -46.6934) (3.574, -46.7049) (3.5468, -46.7164) (3.5194, -46.7276) (3.4919, -46.7387) (3.4644, -46.7496) (3.4367, -46.7604) (3.4089, -46.771) (3.381, -46.7815) (3.3529, -46.7918) (3.3248, -46.802) (3.2966, -46.812) (3.2683, -46.8219) (3.2399, -46.8317) (3.2114, -46.8413) (3.1828, -46.8508) (3.1541, -46.8601) (3.1253, -46.8693) (3.0964, -46.8783) (3.0674, -46.8872) (3.0384, -46.896) (3.0092, -46.9046) (2.98, -46.9131) (2.9507, -46.9215) (2.9213, -46.9297) (2.8918, -46.9378) (2.8622, -46.9457) (2.8326, -46.9536) (2.8028, -46.9613) (2.773, -46.9688) (2.7431, -46.9762) (2.7132, -46.9835) (2.6831, -46.9907) (2.653, -46.9978) (2.6228, -47.0047) (2.5925, -47.0115) (2.5622, -47.0181) (2.5318, -47.0246) (2.5013, -47.031) (2.4707, -47.0373) (2.4401, -47.0434) (2.4094, -47.0495) (2.3848, -47.0542) (2.3663, -47.0577) (2.3539, -47.06) (2.3477, -47.0611) knots 0 0 0 0 0 0 0.01428571 0.02857143 0.04285714 0.05714286 0.07142857 0.08571429 0.1 0.11428571 0.12857143 0.14285714 0.15714286 0.17142857 0.18571429 0.2 0.21428571 0.22857143 0.24285714 0.25714286 0.27142857 0.28571429 0.3 0.31428571 0.32857143 0.34285714 0.35714286 0.37142857 0.38571429 0.4 0.41428571 0.42857143 0.44285714 0.45714286 0.47142857 0.48571429 0.5 0.51428571 0.52857143 0.54285714 0.55714286 0.57142857 0.58571429 0.6 0.61428571 0.62857143 0.64285714 0.65714286 0.67142857 0.68571429 0.7 0.71428571 0.72857143 0.74285714 0.75714286 0.77142857 0.78571429 0.8 0.81428571 0.82857143 0.84285714 0.85714286 0.87142857 0.88571429 0.9 0.91428571 0.92857143 0.94285714 0.95714286 0.97142857 0.98571429 1 1 1 1 1 1
  line L45 (4.2733, -46.306) -> (4.6281, -45.9721)
  arc A91 (4.7688, -45.9757) -> (4.6281, -45.9721) centre (4.6967, -46.0449) ccw
  arc A92 (4.7688, -45.9757) -> (5.5077, -46.6834) centre (13.5, -37.5997) ccw
  arc A93 (5.5174, -46.8238) -> (5.5077, -46.6834) centre (5.4417, -46.7585) ccw
  line L46 (5.5174, -46.8238) -> (5.1991, -47.1927)
  spline S46 degree 5 poles (5.1991, -47.1927) (5.1954, -47.197) (5.1881, -47.2056) (5.1775, -47.2189) (5.164, -47.237) (5.148, -47.2603) (5.1326, -47.2842) (5.1175, -47.3083) (5.1027, -47.3327) (5.0881, -47.3571) (5.0736, -47.3817) (5.0593, -47.4064) (5.0452, -47.4314) (5.0315, -47.4565) (5.018, -47.4819) (5.0048, -47.5075) (4.9919, -47.5333) (4.9792, -47.5593) (4.9667, -47.5854) (4.9544, -47.6116) (4.9422, -47.6379) (4.9302, -47.6644) (4.9184, -47.691) (4.9068, -47.7178) (4.8954, -47.7446) (4.8841, -47.7717) (4.8731, -47.7988) (4.8622, -47.8261) (4.8515, -47.8534) (4.841, -47.8809) (4.8306, -47.9085) (4.8204, -47.9362) (4.8103, -47.9641) (4.8004, -47.992) (4.7907, -48.02) (4.7811, -48.0481) (4.7717, -48.0764) (4.7624, -48.1047) (4.7533, -48.1331) (4.7443, -48.1617) (4.7355, -48.1903) (4.7269, -48.219) (4.7184, -48.2478) (4.71, -48.2767) (4.7018, -48.3057) (4.6937, -48.3347) (4.6858, -48.3639) (4.678, -48.3931) (4.6703, -48.4225) (4.6628, -48.4519) (4.6554, -48.4814) (4.6482, -48.511) (4.6411, -48.5406) (4.6342, -48.5703) (4.6273, -48.6001) (4.6207, -48.63) (4.6141, -48.66) (4.6077, -48.69) (4.6015, -48.7201) (4.5953, -48.7503) (4.5893, -48.7806) (4.5834, -48.8109) (4.5777, -48.8413) (4.5721, -48.8718) (4.5666, -48.9023) (4.5613, -48.9329) (4.5561, -48.9636) (4.551, -48.9943) (4.546, -49.0251) (4.5412, -49.056) (4.5365, -49.0869) (4.5329, -49.1117) (4.5302, -49.1304) (4.5284, -49.1428) (4.5276, -49.149) knots 0 0 0 0 0 0 0.01428571 0.02857143 0.04285714 0.05714286 0.07142857 0.08571429 0.1 0.11428571 0.12857143 0.14285714 0.15714286 0.17142857 0.18571429 0.2 0.21428571 0.22857143 0.24285714 0.25714286 0.27142857 0.28571429 0.3 0.31428571 0.32857143 0.34285714 0.35714286 0.37142857 0.38571429 0.4 0.41428571 0.42857143 0.44285714 0.45714286 0.47142857 0.48571429 0.5 0.51428571 0.52857143 0.54285714 0.55714286 0.57142857 0.58571429 0.6 0.61428571 0.62857143 0.64285714 0.65714286 0.67142857 0.68571429 0.7 0.71428571 0.72857143 0.74285714 0.75714286 0.77142857 0.78571429 0.8 0.81428571 0.82857143 0.84285714 0.85714286 0.87142857 0.88571429 0.9 0.91428571 0.92857143 0.94285714 0.95714286 0.97142857 0.98571429 1 1 1 1 1 1
  arc A94 (4.5276, -49.149) -> (5.1765, -49.6251) centre (13.5, -37.5997) ccw
  spline S47 degree 5 poles (6.8411, -48.3974) (6.8381, -48.4022) (6.832, -48.4117) (6.8226, -48.4258) (6.8093, -48.4441) (6.7919, -48.4664) (6.7738, -48.4883) (6.7552, -48.5098) (6.7365, -48.5313) (6.7175, -48.5526) (6.6984, -48.5738) (6.6791, -48.5949) (6.6596, -48.6158) (6.6397, -48.6365) (6.6195, -48.6569) (6.599, -48.6771) (6.5783, -48.6972) (6.5574, -48.7171) (6.5362, -48.7369) (6.5149, -48.7565) (6.4935, -48.7761) (6.4718, -48.7954) (6.45, -48.8147) (6.428, -48.8338) (6.4057, -48.8528) (6.3833, -48.8716) (6.3608, -48.8903) (6.338, -48.9088) (6.3151, -48.9272) (6.2921, -48.9455) (6.2688, -48.9637) (6.2455, -48.9818) (6.222, -48.9997) (6.1983, -49.0176) (6.1745, -49.0353) (6.1505, -49.0528) (6.1264, -49.0703) (6.1022, -49.0876) (6.0778, -49.1049) (6.0533, -49.122) (6.0286, -49.139) (6.0038, -49.1559) (5.9789, -49.1726) (5.9539, -49.1893) (5.9287, -49.2058) (5.9034, -49.2223) (5.8779, -49.2386) (5.8524, -49.2548) (5.8267, -49.2709) (5.8009, -49.2869) (5.775, -49.3028) (5.7489, -49.3185) (5.7228, -49.3342) (5.6965, -49.3497) (5.6701, -49.3652) (5.6436, -49.3805) (5.617, -49.3958) (5.5903, -49.4109) (5.5634, -49.4259) (5.5365, -49.4408) (5.5094, -49.4556) (5.4823, -49.4703) (5.455, -49.4849) (5.4276, -49.4994) (5.4001, -49.5138) (5.3725, -49.5281) (5.3448, -49.5423) (5.317, -49.5563) (5.2891, -49.5703) (5.2612, -49.5842) (5.2331, -49.5979) (5.2105, -49.6089) (5.1935, -49.617) (5.1822, -49.6224) (5.1765, -49.6251) knots 0 0 0 0 0 0 0.01428571 0.02857143 0.04285714 0.05714286 0.07142857 0.08571429 0.1 0.11428571 0.12857143 0.14285714 0.15714286 0.17142857 0.18571429 0.2 0.21428571 0.22857143 0.24285714 0.25714286 0.27142857 0.28571429 0.3 0.31428571 0.32857143 0.34285714 0.35714286 0.37142857 0.38571429 0.4 0.41428571 0.42857143 0.44285714 0.45714286 0.47142857 0.48571429 0.5 0.51428571 0.52857143 0.54285714 0.55714286 0.57142857 0.58571429 0.6 0.61428571 0.62857143 0.64285714 0.65714286 0.67142857 0.68571429 0.7 0.71428571 0.72857143 0.74285714 0.75714286 0.77142857 0.78571429 0.8 0.81428571 0.82857143 0.84285714 0.85714286 0.87142857 0.88571429 0.9 0.91428571 0.92857143 0.94285714 0.95714286 0.97142857 0.98571429 1 1 1 1 1 1
  line L47 (6.8411, -48.3974) -> (7.0974, -47.983)
  arc A95 (7.2342, -47.9501) -> (7.0974, -47.983) centre (7.1824, -48.0356) ccw
  arc A96 (7.2342, -47.9501) -> (8.1311, -48.4425) centre (13.5, -37.5997) ccw
  line L48 (9.5, -37.5997) -> (9.5, -68.5997)
  arc A97 (9.5, -68.5997) -> (17.5, -68.5997) centre (13.5, -68.5997) ccw
  line L49 (17.5, -68.5997) -> (17.5, -37.5997)
  arc A98 (17.5, -37.5997) -> (9.5, -37.5997) centre (13.5, -37.5997) ccw
  line L50 (13.5, -37.5997) -> (13.5, -68.5997) construction
  circle A99 centre (13.5, -68.5997) radius 1.5
  dimension "d66" = 31
  dimension "d67" = 4
  dimension "d68" = 3
  constraint tangent L48 A97
  constraint tangent A97 L49
  constraint parallel L48 L49
  constraint tangent L49 A98
  constraint tangent L48 A98
  constraint vertical L50
  constraint coincident A0.centre A2.centre
  constraint concentric A97 A99
  measures "d66" distance of A0.centre A97.centre
  measures "d67" radius of A97
  measures "d68" diameter of A99
extrude "Extrude3" add sketch "Sketch5" against normal blind 3 contours S1 L1 A3 A4 A5 L2 S2 A6 S3 L3 A7 A8 A9 L4 S4 A10 S5 L5 A11 A12 A13 L6 L48 L49 A98 | S1 L1 A3 A4 A5 L2 S2 A6 S3 L3 A7 A8 A9 L4 S4 A10 S5 L5 A11 A12 A13 L6 L48 A97 L49 sketch seen with x (0.780061, 0.625704, 0) y (0.625704, -0.780061, 0) z (0, 0, -1) at (-12.9955, 37.7771, 6) bodies 4 in component "Spur Gear (24 teeth)"